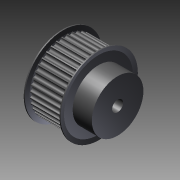
# Autodesk Inventor part: zrr_htd_3m15_6_17034000
Saved by Autodesk Inventor 2011 SP1 (Build 150282100, 282)
## iProperties
Created: 2018-07-07
Part Number: zrr_htd_3m15_6_17034000
Catalog Web Link: www.cadenas.de
Description: zrr_htd_3m15-HTD Pulleys Profile 3M, Timing Belt Width 15mm
Vendor: MAEDLER
Document SubType Name: Modeling
Designer: psAdmin
Manufacturer: MAEDLER
Mass: 72 g
Surface Area: 81.6114 cm^2
Volume: 25.9232 cm^3
Density: 1 g/cm^3
Category: PARTsolutions
Company: MAEDLER
Title: zrr_htd_3m15_6_17034000
Author: Cadenas PARTsolutions
Comments: HTD Pulleys Profile 3M, Timing Belt Width 15mm
PSOL_IDENT_0: {$CADENAS_DATA\23d-libs\maedler\antriebselemente\zahnriemenraeder_zahnriemen\zahnriemenraeder\htd-pr
PSOL_IDENT_1: ofil\zrr_htd_3m15.prj},197 {VTYP=3D},{NB=zrr_htd_3m15_6_17034000},{LINA=zrr_htd_3m15_6_17034000},{NN=
PSOL_IDENT_2: zrr_htd_3m15},{DATE=16.06.2017 10:47:49},{GEOMDATE=09.06.2016 09:07:07},{VERSION=},{LINEID=360},{LIN
PSOL_IDENT_3: ESUBID=-1},{WBVAR=BX}  {NB=zrr_htd_3m15_6_17034000},{LINA=zrr_htd_3m15_6_17034000},{KT=DUMMY},{ARTNR=
PSOL_IDENT_4: 17034000},{PDF=PDF Katalogseite},{AUSF=40-3M-15-1F},{MAT=Aluminium},{ZTL=3.000},{ZRB=15.000},{Z=40.0
PSOL_IDENT_5: 00},{AUS=1F},{ZS=37.440},{BS=42.000},{DO=38.200},{ND=28.000},{B=20.000},{L=30.000},{I=0.000},{VB=6.0
PSOL_IDENT_6: 00},{FB=16.500},{BX=6},{GEW=72.000},{ZT=1.200},{ZB=1.800},{T=1.000},{BB=1.000}
NN: zrr_htd_3m15
NT: HTD-Zahnriemenräder Profil 3M, Zahnriemenbreite 15mm
NB: zrr_htd_3m15_6_17034000
NBSYN: zrr_htd_3m15_$BX._$ARTNR.
LINA: zrr_htd_3m15_6_17034000
ARTNR: 17034000
PDF: PDF Katalogseite
AUSF: 40-3M-15-1F
MAT: Aluminium
ZTL: 3.000
ZRB: 15.000
Z: 40.000
AUS: 1F
ZS: 37.440
BS: 42.000
DO: 38.200
ND: 28.000
B: 20.000
L: 30.000
I: 0.000
VB: 6.000
FB: 16.500
BX: 6
GEW: 72.000
ZT: 1.200
ZB: 1.800
T: 1.000
BB: 1.000
SUPPLIER: MAEDLER
ARTICLENO: zrr_htd_3m15_6_17034000
BOMINFO: zrr_htd_3m15_6_17034000
CREATOR: CADENAS GmbH
Autodesk Inventor part; units mm, degrees
ref_plane "YZ Plane" through (0, 0, 0) normal (1, 0, 0) x (0, 1, 0)
ref_plane "XZ Plane" through (0, 0, 0) normal (0, 1, 0) x (-1, 0, 0)
ref_plane "XY Plane" through (0, 0, 0) normal (0, 0, 1) x (1, 0, 0)
sketch "Sketch_3" plane through (0, 0, 0) normal (0, 0, 1) x (1, 0, 0)
  line L0 (500, 0) -> (-500, 0)
  line L1 (0, 0) -> (0, 21)
  line L2 (0, 21) -> (0.598, 21)
  line L3 (0.598, 21) -> (1, 18.72)
  line L4 (1, 18.72) -> (19, 18.72)
  line L5 (19, 18.72) -> (19.402, 21)
  line L6 (19.402, 21) -> (20, 21)
  line L7 (20, 21) -> (19.598, 18.72)
  line L8 (19.598, 18.72) -> (19.598, 14)
  line L9 (19.598, 14) -> (30, 14)
  line L10 (30, 14) -> (30, 0)
  line L11 (30, 0) -> (0, 0)
  constraints: 24 end point
revolve "Revolution1" add sketch "Sketch_3" angle 360 about axis through (500, 0, 0) along (1, 0, 0)
sketch "Sketch_4" plane through (1, 0, 0) normal (1, 0, 0) x (0, 0, -1)
  circle A0 centre (0, 0) radius 300
  arc A1 (-18.6815, -1.1994) -> (-18.6623, -1.4688) centre (0, 0) ccw
  arc A2 (-18.6623, -1.4688) -> (-18.6392, -1.7378) centre (0, 0) ccw
  arc A3 (-18.2639, -4.1071) -> (-18.6392, -1.7378) centre (-18.4895, -2.9285) ccw
  arc A4 (-18.2639, -4.1071) -> (-18.2028, -4.3701) centre (0, 0) ccw
  arc A5 (-18.2028, -4.3701) -> (-18.1378, -4.6322) centre (0, 0) ccw
  arc A6 (-17.3966, -6.9136) -> (-18.1378, -4.6322) centre (-17.8038, -5.7848) ccw
  arc A7 (-17.3966, -6.9136) -> (-17.295, -7.1638) centre (0, 0) ccw
  arc A8 (-17.295, -7.1638) -> (-17.1899, -7.4126) centre (0, 0) ccw
  arc A9 (-16.1009, -9.5499) -> (-17.1899, -7.4126) centre (-16.6796, -8.4987) ccw
  arc A10 (-16.1009, -9.5499) -> (-15.9614, -9.7812) centre (0, 0) ccw
  arc A11 (-15.9614, -9.7812) -> (-15.8187, -10.0104) centre (0, 0) ccw
  arc A12 (-14.4087, -11.9511) -> (-15.8187, -10.0104) centre (-15.1448, -11.0033) ccw
  arc A13 (-14.4087, -11.9511) -> (-14.2348, -12.1577) centre (0, 0) ccw
  arc A14 (-14.2348, -12.1577) -> (-14.0579, -12.3618) centre (0, 0) ccw
  arc A15 (-12.3618, -14.0579) -> (-14.0579, -12.3618) centre (-13.237, -13.237) ccw
  arc A16 (-12.3618, -14.0579) -> (-12.1577, -14.2348) centre (0, 0) ccw
  arc A17 (-12.1577, -14.2348) -> (-11.9511, -14.4087) centre (0, 0) ccw
  arc A18 (-10.0104, -15.8187) -> (-11.9511, -14.4087) centre (-11.0033, -15.1448) ccw
  arc A19 (-10.0104, -15.8187) -> (-9.7812, -15.9614) centre (0, 0) ccw
  arc A20 (-9.7812, -15.9614) -> (-9.5499, -16.1009) centre (0, 0) ccw
  arc A21 (-7.4126, -17.1899) -> (-9.5499, -16.1009) centre (-8.4987, -16.6796) ccw
  arc A22 (-7.4126, -17.1899) -> (-7.1638, -17.295) centre (0, 0) ccw
  arc A23 (-7.1638, -17.295) -> (-6.9136, -17.3966) centre (0, 0) ccw
  arc A24 (-4.6322, -18.1378) -> (-6.9136, -17.3966) centre (-5.7848, -17.8038) ccw
  arc A25 (-4.6322, -18.1378) -> (-4.3701, -18.2028) centre (0, 0) ccw
  arc A26 (-4.3701, -18.2028) -> (-4.1071, -18.2639) centre (0, 0) ccw
  arc A27 (-1.7378, -18.6392) -> (-4.1071, -18.2639) centre (-2.9285, -18.4895) ccw
  arc A28 (-1.7378, -18.6392) -> (-1.4688, -18.6623) centre (0, 0) ccw
  arc A29 (-1.4688, -18.6623) -> (-1.1994, -18.6815) centre (0, 0) ccw
  arc A30 (1.1994, -18.6815) -> (-1.1994, -18.6815) centre (0, -18.72) ccw
  arc A31 (1.1994, -18.6815) -> (1.4688, -18.6623) centre (0, 0) ccw
  arc A32 (1.4688, -18.6623) -> (1.7378, -18.6392) centre (0, 0) ccw
  arc A33 (4.1071, -18.2639) -> (1.7378, -18.6392) centre (2.9285, -18.4895) ccw
  arc A34 (4.1071, -18.2639) -> (4.3701, -18.2028) centre (0, 0) ccw
  arc A35 (4.3701, -18.2028) -> (4.6322, -18.1378) centre (0, 0) ccw
  arc A36 (6.9136, -17.3966) -> (4.6322, -18.1378) centre (5.7848, -17.8038) ccw
  arc A37 (6.9136, -17.3966) -> (7.1638, -17.295) centre (0, 0) ccw
  arc A38 (7.1638, -17.295) -> (7.4126, -17.1899) centre (0, 0) ccw
  arc A39 (9.5499, -16.1009) -> (7.4126, -17.1899) centre (8.4987, -16.6796) ccw
  arc A40 (9.5499, -16.1009) -> (9.7812, -15.9614) centre (0, 0) ccw
  arc A41 (9.7812, -15.9614) -> (10.0104, -15.8187) centre (0, 0) ccw
  arc A42 (11.9511, -14.4087) -> (10.0104, -15.8187) centre (11.0033, -15.1448) ccw
  arc A43 (11.9511, -14.4087) -> (12.1577, -14.2348) centre (0, 0) ccw
  arc A44 (12.1577, -14.2348) -> (12.3618, -14.0579) centre (0, 0) ccw
  arc A45 (14.0579, -12.3618) -> (12.3618, -14.0579) centre (13.237, -13.237) ccw
  arc A46 (14.0579, -12.3618) -> (14.2348, -12.1577) centre (0, 0) ccw
  arc A47 (14.2348, -12.1577) -> (14.4087, -11.9511) centre (0, 0) ccw
  arc A48 (15.8187, -10.0104) -> (14.4087, -11.9511) centre (15.1448, -11.0033) ccw
  arc A49 (15.8187, -10.0104) -> (15.9614, -9.7812) centre (0, 0) ccw
  arc A50 (15.9614, -9.7812) -> (16.1009, -9.5499) centre (0, 0) ccw
  arc A51 (17.1899, -7.4126) -> (16.1009, -9.5499) centre (16.6796, -8.4987) ccw
  arc A52 (17.1899, -7.4126) -> (17.295, -7.1638) centre (0, 0) ccw
  arc A53 (17.295, -7.1638) -> (17.3966, -6.9136) centre (0, 0) ccw
  arc A54 (18.1378, -4.6322) -> (17.3966, -6.9136) centre (17.8038, -5.7848) ccw
  arc A55 (18.1378, -4.6322) -> (18.2028, -4.3701) centre (0, 0) ccw
  arc A56 (18.2028, -4.3701) -> (18.2639, -4.1071) centre (0, 0) ccw
  arc A57 (18.6392, -1.7378) -> (18.2639, -4.1071) centre (18.4895, -2.9285) ccw
  arc A58 (18.6392, -1.7378) -> (18.6623, -1.4688) centre (0, 0) ccw
  arc A59 (18.6623, -1.4688) -> (18.6815, -1.1994) centre (0, 0) ccw
  arc A60 (18.6815, 1.1994) -> (18.6815, -1.1994) centre (18.72, 0) ccw
  arc A61 (18.6815, 1.1994) -> (18.6623, 1.4688) centre (0, 0) ccw
  arc A62 (18.6623, 1.4688) -> (18.6392, 1.7378) centre (0, 0) ccw
  arc A63 (18.2639, 4.1071) -> (18.6392, 1.7378) centre (18.4895, 2.9285) ccw
  arc A64 (18.2639, 4.1071) -> (18.2028, 4.3701) centre (0, 0) ccw
  arc A65 (18.2028, 4.3701) -> (18.1378, 4.6322) centre (0, 0) ccw
  arc A66 (17.3966, 6.9136) -> (18.1378, 4.6322) centre (17.8038, 5.7848) ccw
  arc A67 (17.3966, 6.9136) -> (17.295, 7.1638) centre (0, 0) ccw
  arc A68 (17.295, 7.1638) -> (17.1899, 7.4126) centre (0, 0) ccw
  arc A69 (16.1009, 9.5499) -> (17.1899, 7.4126) centre (16.6796, 8.4987) ccw
  arc A70 (16.1009, 9.5499) -> (15.9614, 9.7812) centre (0, 0) ccw
  arc A71 (15.9614, 9.7812) -> (15.8187, 10.0104) centre (0, 0) ccw
  arc A72 (14.4087, 11.9511) -> (15.8187, 10.0104) centre (15.1448, 11.0033) ccw
  arc A73 (14.4087, 11.9511) -> (14.2348, 12.1577) centre (0, 0) ccw
  arc A74 (14.2348, 12.1577) -> (14.0579, 12.3618) centre (0, 0) ccw
  arc A75 (12.3618, 14.0579) -> (14.0579, 12.3618) centre (13.237, 13.237) ccw
  arc A76 (12.3618, 14.0579) -> (12.1577, 14.2348) centre (0, 0) ccw
  arc A77 (12.1577, 14.2348) -> (11.9511, 14.4087) centre (0, 0) ccw
  arc A78 (10.0104, 15.8187) -> (11.9511, 14.4087) centre (11.0033, 15.1448) ccw
  arc A79 (10.0104, 15.8187) -> (9.7812, 15.9614) centre (0, 0) ccw
  arc A80 (9.7812, 15.9614) -> (9.5499, 16.1009) centre (0, 0) ccw
  arc A81 (7.4126, 17.1899) -> (9.5499, 16.1009) centre (8.4987, 16.6796) ccw
  arc A82 (7.4126, 17.1899) -> (7.1638, 17.295) centre (0, 0) ccw
  arc A83 (7.1638, 17.295) -> (6.9136, 17.3966) centre (0, 0) ccw
  arc A84 (4.6322, 18.1378) -> (6.9136, 17.3966) centre (5.7848, 17.8038) ccw
  arc A85 (4.6322, 18.1378) -> (4.3701, 18.2028) centre (0, 0) ccw
  arc A86 (4.3701, 18.2028) -> (4.1071, 18.2639) centre (0, 0) ccw
  arc A87 (1.7378, 18.6392) -> (4.1071, 18.2639) centre (2.9285, 18.4895) ccw
  arc A88 (1.7378, 18.6392) -> (1.4688, 18.6623) centre (0, 0) ccw
  arc A89 (1.4688, 18.6623) -> (1.1994, 18.6815) centre (0, 0) ccw
  arc A90 (-1.1994, 18.6815) -> (1.1994, 18.6815) centre (0, 18.72) ccw
  arc A91 (-1.1994, 18.6815) -> (-1.4688, 18.6623) centre (0, 0) ccw
  arc A92 (-1.4688, 18.6623) -> (-1.7378, 18.6392) centre (0, 0) ccw
  arc A93 (-4.1071, 18.2639) -> (-1.7378, 18.6392) centre (-2.9285, 18.4895) ccw
  arc A94 (-4.1071, 18.2639) -> (-4.3701, 18.2028) centre (0, 0) ccw
  arc A95 (-4.3701, 18.2028) -> (-4.6322, 18.1378) centre (0, 0) ccw
  arc A96 (-6.9136, 17.3966) -> (-4.6322, 18.1378) centre (-5.7848, 17.8038) ccw
  arc A97 (-6.9136, 17.3966) -> (-7.1638, 17.295) centre (0, 0) ccw
  arc A98 (-7.1638, 17.295) -> (-7.4126, 17.1899) centre (0, 0) ccw
  arc A99 (-9.5499, 16.1009) -> (-7.4126, 17.1899) centre (-8.4987, 16.6796) ccw
  arc A100 (-9.5499, 16.1009) -> (-9.7812, 15.9614) centre (0, 0) ccw
  arc A101 (-9.7812, 15.9614) -> (-10.0104, 15.8187) centre (0, 0) ccw
  arc A102 (-11.9511, 14.4087) -> (-10.0104, 15.8187) centre (-11.0033, 15.1448) ccw
  arc A103 (-11.9511, 14.4087) -> (-12.1577, 14.2348) centre (0, 0) ccw
  arc A104 (-12.1577, 14.2348) -> (-12.3618, 14.0579) centre (0, 0) ccw
  arc A105 (-14.0579, 12.3618) -> (-12.3618, 14.0579) centre (-13.237, 13.237) ccw
  arc A106 (-14.0579, 12.3618) -> (-14.2348, 12.1577) centre (0, 0) ccw
  arc A107 (-14.2348, 12.1577) -> (-14.4087, 11.9511) centre (0, 0) ccw
  arc A108 (-15.8187, 10.0104) -> (-14.4087, 11.9511) centre (-15.1448, 11.0033) ccw
  arc A109 (-15.8187, 10.0104) -> (-15.9614, 9.7812) centre (0, 0) ccw
  arc A110 (-15.9614, 9.7812) -> (-16.1009, 9.5499) centre (0, 0) ccw
  arc A111 (-17.1899, 7.4126) -> (-16.1009, 9.5499) centre (-16.6796, 8.4987) ccw
  arc A112 (-17.1899, 7.4126) -> (-17.295, 7.1638) centre (0, 0) ccw
  arc A113 (-17.295, 7.1638) -> (-17.3966, 6.9136) centre (0, 0) ccw
  arc A114 (-18.1378, 4.6322) -> (-17.3966, 6.9136) centre (-17.8038, 5.7848) ccw
  arc A115 (-18.1378, 4.6322) -> (-18.2028, 4.3701) centre (0, 0) ccw
  arc A116 (-18.2028, 4.3701) -> (-18.2639, 4.1071) centre (0, 0) ccw
  arc A117 (-18.6392, 1.7378) -> (-18.2639, 4.1071) centre (-18.4895, 2.9285) ccw
  arc A118 (-18.6392, 1.7378) -> (-18.6623, 1.4688) centre (0, 0) ccw
  arc A119 (-18.6623, 1.4688) -> (-18.6815, 1.1994) centre (0, 0) ccw
  arc A120 (-18.6815, -1.1994) -> (-18.6815, 1.1994) centre (-18.72, 0) ccw
  constraints: 240 point on circle, 121 centre point
extrude "Extrusion1" cut sketch "Sketch_4" along normal blind 18
sketch "Sketch_9_ALT_Drilling_1" plane through (0, 0, 0) normal (1, 0, 0) x (0, 1, 0)
  circle A0 centre (0, 0) radius 3
  constraints: 1 centre point
extrude "Extrusion2" cut sketch "Sketch_9_ALT_Drilling_1" along normal blind 30
body "Solid1"
